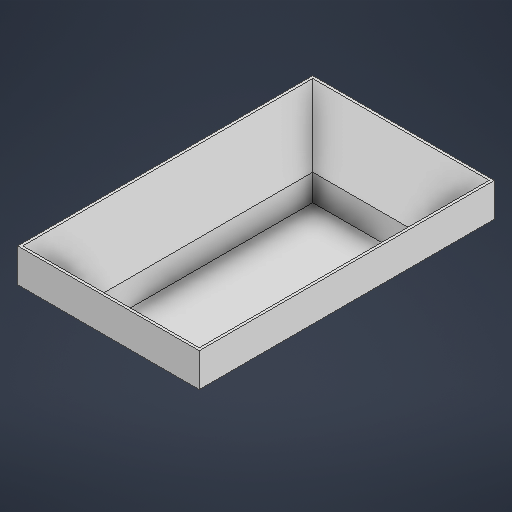
# Autodesk Inventor part: мыльница
Saved by Autodesk Inventor 2025 (Build 290162000, 162)
## iProperties
Created: 2024-12-03
Part Number: мыльница
Material: Типовые
Document SubType Name: Modeling
Designer: GameHD
Density: 1 g/cm^3
Appearance: По умолчанию
Author: GameHD
Autodesk Inventor part; units mm, degrees
ref_plane "YZ Plane" through (0, 0, 0) normal (1, 0, 0) x (0, 1, 0)
ref_plane "XZ Plane" through (0, 0, 0) normal (0, 1, 0) x (-1, 0, 0)
ref_plane "XY Plane" through (0, 0, 0) normal (0, 0, 1) x (1, 0, 0)
sketch "Эскиз1" plane through (0, 0, 0) normal (0, 0, 1) x (1, 0, 0)
  line L0 (-19.75, -19.75) -> (19.75, -19.75)
  line L1 (19.75, -19.75) -> (19.75, 19.75)
  line L2 (19.75, 19.75) -> (-19.75, 19.75)
  line L3 (-19.75, 19.75) -> (-19.75, -19.75)
  line L4 (-19.75, -19.75) -> (19.75, 19.75) construction
  line L5 (19.75, -19.75) -> (-19.75, 19.75) construction
  line L6 (-40, -40) -> (40, -40)
  line L7 (40, -40) -> (40, 40)
  line L8 (40, 40) -> (-40, 40)
  line L9 (-40, 40) -> (-40, -40)
  line L10 (-40, -40) -> (40, 40) construction
  line L11 (40, -40) -> (-40, 40) construction
  line L12 (-19.75, 19.75) -> (-40, 19.75)
  line L13 (19.75, 19.75) -> (40, 19.75)
  point P0 (0, 0)
  dimension "d0" = 39.5
  dimension "d1" = 39.5
  dimension "d2" = 80
  dimension "d3" = 80
  constraints: 28 end point, 4 midpoint, 4 parallel, 3 perpendicular, 3 point on line, 2 horizontal
  measures "d0" distance of L2.end L1.end
  measures "d1" distance of L1.end L0.end
  measures "d2" distance of L8.end L7.end
  measures "d3" distance of L8.end L6.start
extrude "Выдавливание1" add sketch "Эскиз1" along normal blind 92 contours L0 L1 L13 L7 L6 L9 L12 L3
sketch "Эскиз2" plane through (0, 0, 0) normal (0, 0, -1) x (-1, 0, 0)
  line L0 (-19.75, -19.75) -> (19.75, -19.75) projected
  line L1 (-19.75, 19.75) -> (-19.75, -19.75) projected
  line L2 (-40, 19.75) -> (-19.75, 19.75) projected
  line L3 (-40, -40) -> (-40, 19.75) projected
  line L4 (40, -40) -> (-40, -40) projected
  line L5 (40, 19.75) -> (40, -40) projected
  line L6 (19.75, 19.75) -> (40, 19.75) projected
  line L7 (19.75, -19.75) -> (19.75, 19.75) projected
  line L8 (-19.75, 19.75) -> (19.75, 19.75)
  point P0 (0, 0)
  constraints: 2 end point, 1 horizontal
extrude "Выдавливание2" add sketch "Эскиз2" along normal blind 19
sketch "Эскиз3" plane through (0, 0, 92) normal (0, 0, 1) x (1, 0, 0)
  line L0 (19.75, -19.75) -> (-19.75, -19.75) projected
  line L1 (-19.75, -19.75) -> (-19.75, 19.75) projected
  line L2 (-19.75, 19.75) -> (-40, 19.75) projected
  line L3 (-40, 19.75) -> (-40, -40) projected
  line L4 (-40, -40) -> (40, -40) projected
  line L5 (40, -40) -> (40, 19.75) projected
  line L6 (40, 19.75) -> (19.75, 19.75) projected
  line L7 (19.75, 19.75) -> (19.75, -19.75) projected
  line L8 (-19.75, 19.75) -> (19.75, 19.75) projected
  point P0 (0, 0)
extrude "Выдавливание3" add sketch "Эскиз3" along normal blind 19
sketch "Эскиз4" plane through (-40, -40, -19) normal (-1, 0, 0) x (0, 0, 1)
  line L0 (0, 59.75) -> (200, 59.75)
  line L1 (200, 59.75) -> (200, 49.75)
  line L2 (200, 49.75) -> (0, 49.75)
  line L3 (0, 49.75) -> (0, 59.75)
  dimension "d12" = 200
  dimension "d13" = 10
  constraints: 8 end point, 2 parallel, 1 horizontal, 1 perpendicular
  measures "d12" distance of L1.end L2.end
  measures "d13" distance of L0.end L1.end
extrude "Выдавливание4" cut sketch "Эскиз4" against normal through all
sketch "Эскиз5" plane through (-40, -40, -19) normal (0, -1, 0) x (1, 0, 0)
  line L0 (80, 0) -> (80, 130) projected
  line L1 (0, 130) -> (80, 130) projected
  line L2 (0, 0) -> (0, 130) projected
  line L3 (80, 0) -> (0, 0) projected
  point P0 (40, 19)
extrude "Выдавливание5" cut sketch "Эскиз5" against normal blind 17.05
sketch "Эскиз6" plane through (-19.75, -19.75, 0) normal (0, 1, 0) x (1, 0, 0)
  line L0 (39.5, 0) -> (0, 0) projected
  line L1 (0, 0) -> (0, -92) projected
  line L2 (39.5, -92) -> (0, -92) projected
  line L3 (39.5, 0) -> (39.5, -92) projected
  line L4 (-1.25, -92) -> (-1.25, 0)
  line L5 (-1.25, 0) -> (40.75, 0)
  line L6 (40.75, 0) -> (40.75, -92)
  line L7 (40.75, -92) -> (-1.25, -92)
  line L8 (-1.25, -92) -> (40.75, 0) construction
  line L9 (-1.25, 0) -> (40.75, -92) construction
  point P0 (19.75, 0)
  point P1 (19.75, -46)
  dimension "d22" = 42
  constraints: 12 end point, 2 midpoint, 2 parallel, 2 perpendicular
  measures "d22" distance of L4.end L5.end
extrude "Выдавливание6" cut sketch "Эскиз6" along normal through all
chamfer "Фаска5" distance 17.875 angle 45 4 edges at (0, 9.75, 92) (21, 9.75, 46) (-21, 9.75, 46) (0, 9.75, 0)
chamfer "Фаска6" distance 17.875 angle 45 4 edges at (-40, -22.95, 46) (0, -22.95, -19) (40, -22.95, 46) (0, -22.95, 111)
